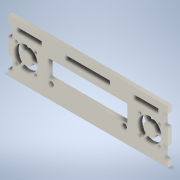
# Autodesk Inventor part: case bottom back
Saved by Autodesk Inventor 2022.2 (Build 262287010, 287A)
## iProperties
Created: 2021-05-28
Part Number: case bottom back
Material: Titanium
Document SubType Name: Modeling
Designer: benka
Density: 4.51 g/cm^3
Appearance: Titanium
Author: benka
Autodesk Inventor part; units mm, degrees
ref_plane "YZ Plane" through (0, 0, 0) normal (1, 0, 0) x (0, 1, 0)
ref_plane "XZ Plane" through (0, 0, 0) normal (0, 1, 0) x (-1, 0, 0)
ref_plane "XY Plane" through (0, 0, 0) normal (0, 0, 1) x (1, 0, 0)
sketch "Sketch1" plane through (0, 0, 0) normal (0, 0, 1) x (1, 0, 0)
  circle A0 centre (45.5, -15.3826) radius 3
  circle A1 centre (-45.5, -15.3826) radius 3
  line L0 (44.6636, 0.7689) -> (35.6636, 0.7689)
  line L1 (33.6636, 2.7689) -> (33.6636, 5.2689)
  line L2 (46.6636, 5.2689) -> (46.6636, 2.7689)
  line L3 (29.9455, -2.1666) -> (-2.0545, -2.1666)
  line L4 (-4.0545, -0.1666) -> (-4.0545, 2.8334)
  line L5 (31.9455, 2.8334) -> (31.9455, -0.1666)
  circle A2 centre (89.024, -15.4039) radius 1.5
  circle A3 centre (65.024, -15.4039) radius 1.5
  circle A4 centre (89.024, 8.5961) radius 1.5
  circle A5 centre (65.024, 8.5961) radius 1.5
  arc A6 (67.8322, 7.6809) -> (67.8322, -14.4886) centre (77.024, -3.4039) ccw
  line L6 (69.3366, 7.4111) -> (71.8641, 3.0334)
  arc A7 (71.8641, 3.0334) -> (71.8641, -9.8411) centre (77.024, -3.4039) ccw
  line L7 (71.8641, -9.8411) -> (69.3366, -14.2188)
  arc A8 (67.8322, -14.4886) -> (69.3366, -14.2188) centre (68.4705, -13.7188) ccw
  arc A9 (69.3366, 7.4111) -> (67.8322, 7.6809) centre (68.4705, 6.9111) ccw
  arc A10 (91.2195, -0.986) -> (72.0202, 10.0988) centre (77.024, -3.4039) ccw
  arc A11 (72.0202, 10.0988) -> (71.5016, 8.6611) centre (72.3677, 9.1611) ccw
  line L8 (74.0291, 4.2834) -> (71.5016, 8.6611)
  arc A12 (85.1787, -2.1539) -> (74.0291, 4.2834) centre (77.024, -3.4039) ccw
  line L9 (90.2337, -2.1539) -> (85.1787, -2.1539)
  arc A13 (90.2337, -2.1539) -> (91.2195, -0.986) centre (90.2337, -1.1539) ccw
  line L10 (85.1787, -4.6539) -> (90.2337, -4.6539)
  arc A14 (91.2195, -5.8218) -> (90.2337, -4.6539) centre (90.2337, -5.6539) ccw
  arc A15 (72.0202, -16.9065) -> (91.2195, -5.8218) centre (77.024, -3.4039) ccw
  arc A16 (71.5016, -15.4688) -> (72.0202, -16.9065) centre (72.3677, -15.9688) ccw
  line L11 (71.5016, -15.4688) -> (74.0291, -11.0911)
  arc A17 (74.0291, -11.0911) -> (85.1787, -4.6539) centre (77.024, -3.4039) ccw
  circle A18 centre (-64.8953, -15.374) radius 1.5
  circle A19 centre (-88.8953, -15.374) radius 1.5
  circle A20 centre (-88.8953, 8.626) radius 1.5
  circle A21 centre (-64.8953, 8.626) radius 1.5
  arc A22 (-62.6997, -0.956) -> (-81.8991, 10.1287) centre (-76.8953, -3.374) ccw
  arc A23 (-81.8991, 10.1287) -> (-82.4176, 8.691) centre (-81.5516, 9.191) ccw
  line L12 (-79.8901, 4.3133) -> (-82.4176, 8.691)
  line L13 (-84.5827, 7.441) -> (-82.0552, 3.0633)
  arc A24 (-84.5827, 7.441) -> (-86.087, 7.7108) centre (-85.4487, 6.941) ccw
  arc A25 (-86.087, 7.7108) -> (-86.087, -14.4587) centre (-76.8953, -3.374) ccw
  arc A26 (-82.0552, 3.0633) -> (-82.0552, -9.8112) centre (-76.8953, -3.374) ccw
  arc A27 (-68.7405, -2.124) -> (-79.8901, 4.3133) centre (-76.8953, -3.374) ccw
  line L14 (-63.6855, -2.124) -> (-68.7405, -2.124)
  arc A28 (-63.6855, -2.124) -> (-62.6997, -0.956) centre (-63.6855, -1.124) ccw
  line L15 (-68.7405, -4.624) -> (-63.6855, -4.624)
  arc A29 (-62.6997, -5.7919) -> (-63.6855, -4.624) centre (-63.6855, -5.624) ccw
  arc A30 (-81.8991, -16.8766) -> (-62.6997, -5.7919) centre (-76.8953, -3.374) ccw
  arc A31 (-79.8901, -11.0612) -> (-68.7405, -4.624) centre (-76.8953, -3.374) ccw
  line L16 (-82.4176, -15.4389) -> (-79.8901, -11.0612)
  arc A32 (-82.4176, -15.4389) -> (-81.8991, -16.8766) centre (-81.5516, -15.9389) ccw
  line L17 (-82.0552, -9.8112) -> (-84.5827, -14.1889)
  arc A33 (-86.087, -14.4587) -> (-84.5827, -14.1889) centre (-85.4487, -13.6889) ccw
  line L18 (-2.0545, 4.8334) -> (29.9455, 4.8334)
  line L19 (35.6636, 7.2689) -> (44.6636, 7.2689)
  arc A34 (-4.0545, -0.1666) -> (-2.0545, -2.1666) centre (-2.0545, -0.1666) ccw
  arc A35 (-2.0545, 4.8334) -> (-4.0545, 2.8334) centre (-2.0545, 2.8334) ccw
  arc A36 (31.9455, 2.8334) -> (29.9455, 4.8334) centre (29.9455, 2.8334) ccw
  arc A37 (29.9455, -2.1666) -> (31.9455, -0.1666) centre (29.9455, -0.1666) ccw
  arc A38 (33.6636, 2.7689) -> (35.6636, 0.7689) centre (35.6636, 2.7689) ccw
  arc A39 (35.6636, 7.2689) -> (33.6636, 5.2689) centre (35.6636, 5.2689) ccw
  arc A40 (46.6636, 5.2689) -> (44.6636, 7.2689) centre (44.6636, 5.2689) ccw
  arc A41 (44.6636, 0.7689) -> (46.6636, 2.7689) centre (44.6636, 2.7689) ccw
  line L20 (-87.4504, 24.6174) -> (-57.4504, 24.6174)
  line L21 (-87.4504, 19.6174) -> (-87.4504, 24.6174)
  line L22 (-87.4504, 19.6174) -> (-57.4504, 19.6174)
  line L23 (-57.4504, 19.6174) -> (-57.4504, 24.6174)
  line L24 (-27.4504, 19.6174) -> (27.5496, 19.6174)
  line L25 (27.5496, 19.6174) -> (27.5496, 24.6174)
  line L26 (-27.4504, 24.6174) -> (27.5496, 24.6174)
  line L27 (-27.4504, 19.6174) -> (-27.4504, 24.6174)
  line L28 (57.5496, 19.6174) -> (87.5496, 19.6174)
  line L29 (87.5496, 19.6174) -> (87.5496, 24.6174)
  line L30 (57.5496, 24.6174) -> (87.5496, 24.6174)
  line L31 (57.5496, 19.6174) -> (57.5496, 24.6174)
  line L32 (-98.9504, -25.3833) -> (-98.9504, -33.3826)
  line L33 (99.0496, -33.3826) -> (-98.9504, -33.3826)
  line L34 (-98.9504, 24.6174) -> (-93.9504, 24.6174)
  line L35 (-93.9504, 24.6174) -> (-93.9504, 9.6159)
  line L36 (-98.9504, 9.6159) -> (-93.9504, 9.6159)
  line L37 (-98.9504, 9.6159) -> (-98.9504, -10.3841)
  line L38 (-98.9504, -10.3841) -> (-93.9504, -10.3841)
  line L39 (-93.9504, -10.3841) -> (-93.9504, -25.3833)
  line L40 (-98.9504, -25.3833) -> (-93.9504, -25.3833)
  line L41 (99.0496, -25.3833) -> (99.0496, -33.3833)
  line L42 (94.0496, -25.3833) -> (99.0496, -25.3833)
  line L43 (94.0496, -10.3841) -> (94.0496, -25.3833)
  line L44 (94.0496, -10.3841) -> (99.0496, -10.3841)
  line L45 (99.0496, 9.6159) -> (99.0496, -10.3841)
  line L46 (94.0496, 9.6159) -> (99.0496, 9.6159)
  line L47 (94.0496, 24.6174) -> (94.0496, 9.6159)
  line L48 (94.0496, 24.6174) -> (99.0496, 24.6174)
  line L49 (-98.9504, 24.6174) -> (-98.9504, 32.6174)
  line L50 (-98.9504, 32.6174) -> (99.0496, 32.6174)
  line L51 (99.0496, 32.6174) -> (99.0496, 24.6174)
  line L52 (-22.6436, -2.2792) -> (-22.6436, -8.2792)
  line L53 (-35.6436, -0.2792) -> (-24.6436, -0.2792)
  line L54 (-24.6436, -10.2792) -> (-35.6436, -10.2792)
  line L55 (-37.6436, -8.2792) -> (-37.6436, -2.2792)
  arc A42 (-35.6436, -0.2792) -> (-37.6436, -2.2792) centre (-35.6436, -2.2792) ccw
  arc A43 (-22.6436, -2.2792) -> (-24.6436, -0.2792) centre (-24.6436, -2.2792) ccw
  arc A44 (-24.6436, -10.2792) -> (-22.6436, -8.2792) centre (-24.6436, -8.2792) ccw
  arc A45 (-37.6436, -8.2792) -> (-35.6436, -10.2792) centre (-35.6436, -8.2792) ccw
  line L56 (-5.5869, 3.8805) -> (-5.5869, -1.877)
  line L57 (-7.5869, -3.877) -> (-13.5192, -3.877)
  line L58 (-15.5192, -1.877) -> (-15.5192, 3.8805)
  line L59 (-13.5192, 5.8805) -> (-7.5869, 5.8805)
  arc A46 (-13.5192, 5.8805) -> (-15.5192, 3.8805) centre (-13.5192, 3.8805) ccw
  arc A47 (-15.5192, -1.877) -> (-13.5192, -3.877) centre (-13.5192, -1.877) ccw
  arc A48 (-5.5869, 3.8805) -> (-7.5869, 5.8805) centre (-7.5869, 3.8805) ccw
  arc A49 (-7.5869, -3.877) -> (-5.5869, -1.877) centre (-7.5869, -1.877) ccw
  point P0 (-90.9348, -30.6649)
  point P1 (27.5, 24.6174)
  point P2 (0, 0)
  point P3 (-22.6436, -0.2792)
  point P4 (-22.6436, -10.2792)
  point P5 (-37.6436, -0.2792)
  point P6 (-37.6436, -10.2792)
  point P7 (-2.0545, 2.8334)
  dimension "d22" = 91
  dimension "d27" = 7
  dimension "d28" = 36
  dimension "d29" = 13
  dimension "d30" = 6.5
  dimension "d35" = 18
  dimension "d36" = 18
  dimension "d37" = 66
  dimension "d38" = 45.5
  dimension "d39" = 6
  dimension "d40" = 6
  dimension "d41" = 198
  constraints: 122 end point, 80 point on circle, 50 centre point, 32 tangent, 14 equal radius, 10 horizontal, 9 point on line, 8 vertical, 6 parallel, 5 perpendicular, 19 other
  measures "d22" distance of A0.centre A1.centre
  measures "d27" distance between parallel lines of L18 L3
  measures "d28" distance between parallel lines of L5 L4
  measures "d29" distance between parallel lines of L2 L1
  measures "d30" distance between parallel lines of L0 L19
  measures "d35" distance from line of A1.centre L33
  measures "d36" distance from line of L33 A0.centre
  measures "d37" distance between parallel lines of L33 L50
  measures "d38" horizontal distance of point (0, 0) A0.centre
  measures "d39" diameter of A0
  measures "d40" diameter of A1
  measures "d41" distance between parallel lines of L51 L49
extrude "Extrusion1" add sketch "Sketch1" along normal blind 5
sketch "Sketch2" plane through (0, 0, 5) normal (0, 0, 1) x (1, 0, 0)
  line L0 (-44.5, 11.026) -> (44.5, 11.026)
  line L1 (48.5, 7.026) -> (48.5, -6.974)
  line L2 (44.5, -10.974) -> (-44.5, -10.974)
  line L3 (-48.5, -6.974) -> (-48.5, 7.026)
  arc A0 (-44.5, 11.026) -> (-48.5, 7.026) centre (-44.5, 7.026) ccw
  arc A1 (48.5, 7.026) -> (44.5, 11.026) centre (44.5, 7.026) ccw
  arc A2 (44.5, -10.974) -> (48.5, -6.974) centre (44.5, -6.974) ccw
  arc A3 (-48.5, -6.974) -> (-44.5, -10.974) centre (-44.5, -6.974) ccw
  line L4 (99.0496, -10.3841) -> (99.0496, 9.6159) projected
  line L5 (-98.9504, -33.3826) -> (99.0496, -33.3826) projected
  circle A4 centre (-45.5, -15.3826) radius 3 projected
  circle A5 centre (45.5, -15.3826) radius 3 projected
  arc A6 (-62.6997, -0.956) -> (-81.8991, 10.1287) centre (-76.8953, -3.374) ccw projected
  point P0 (0, 0)
  point P1 (-76.8953, -3.374)
  dimension "d48" = 4
  dimension "d58" = 97
  dimension "d59" = 22
  dimension "d60" = 50.5496
  dimension "d61" = 22.4087
  constraints: 11 tangent, 8 end point, 8 point on circle, 4 centre point, 3 equal radius, 2 parallel, 1 horizontal, 1 perpendicular
  measures "d48" radius of A0
  measures "d58" distance between parallel lines of L1 L3
  measures "d59" distance between parallel lines of L2 L0
  measures "d60" distance between parallel lines of L4 L1
  measures "d61" distance between parallel lines of L5 L2
extrude "Extrusion2" cut sketch "Sketch2" against normal up to next contours L0 A1 L1 A2 L2 A3 L3 A0
sketch "Sketch3" plane through (0, 0, 5) normal (0, 0, 1) x (1, 0, 0)
  line L0 (-92.421, 12.1859) -> (-62.2986, 12.1859)
  line L1 (-62.2986, 12.1859) -> (-62.2986, -19.0319)
  line L2 (-62.2986, -19.0319) -> (-92.421, -19.0319)
  line L3 (-92.421, -19.0319) -> (-92.421, 12.1859)
  line L4 (-92.421, 12.1859) -> (-62.2986, -19.0319) construction
  line L5 (-62.2986, 12.1859) -> (-92.421, -19.0319) construction
  line L6 (62.2986, 11.0377) -> (92.6949, 11.0377)
  line L7 (92.6949, 11.0377) -> (92.6949, -17.8837)
  line L8 (92.6949, -17.8837) -> (62.2986, -17.8837)
  line L9 (62.2986, -17.8837) -> (62.2986, 11.0377)
  line L10 (62.2986, 11.0377) -> (92.6949, -17.8837) construction
  line L11 (92.6949, 11.0377) -> (62.2986, -17.8837) construction
  point P0 (0, 0)
  point P1 (-77.3598, -3.423)
  point P2 (77.4968, -3.423)
  constraints: 24 end point, 4 midpoint, 4 parallel, 2 horizontal, 2 perpendicular
extrude "Extrusion3" add sketch "Sketch3" against normal blind 10
body "Solid1"
